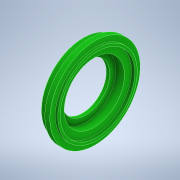
# Autodesk Inventor part: Крышка_Левая
Saved by Autodesk Inventor 2021 (Build 250183000, 183)
## iProperties
Created: 2023-04-24
Part Number: Крышка_Левая
Material: Сталь, углеродистая
Document SubType Name: Modeling
Designer: gdevc
Density: 7.85 g/cm^3
Appearance: Темно-зеленый
Author: gdevc
Autodesk Inventor part; units mm, degrees
ref_plane "YZ Plane" through (0, 0, 0) normal (1, 0, 0) x (0, 1, 0)
ref_plane "XZ Plane" through (0, 0, 0) normal (0, 1, 0) x (-1, 0, 0)
ref_plane "XY Plane" through (0, 0, 0) normal (0, 0, 1) x (1, 0, 0)
sketch "Эскиз1" plane through (0, 0, 0) normal (0, 0, 1) x (1, 0, 0)
  line L0 (0, 0) -> (118.4333, 0)
  line L1 (0, 28.5) -> (4, 28.5)
  line L2 (4, 28.5) -> (4, 36)
  line L3 (0, 28.5) -> (0, 50)
  line L4 (0, 50) -> (9, 50)
  line L5 (9, 50) -> (9, 54)
  line L6 (9, 54) -> (15, 54)
  line L7 (15, 54) -> (15, 47.5)
  line L8 (4, 36) -> (12, 36)
  line L9 (15, 47.5) -> (18, 47.5)
  line L10 (18, 47.5) -> (18, 44.5)
  line L11 (18, 44.5) -> (14.1429, 44.5)
  line L12 (14.1429, 44.5) -> (14.1429, 36)
  line L13 (14.1429, 36) -> (12, 36)
  dimension "d0" = 57
  dimension "d1" = 100
  dimension "d3" = 6
  dimension "d4" = 4
  dimension "d6" = 72
  dimension "d7" = 8
  dimension "d8" = 4
  dimension "d10" = 3
  dimension "d11" = 95
  dimension "d13" = 9
  dimension "d17" = 3
  constraints: 28 end point, 6 perpendicular, 4 horizontal, 2 vertical, 1 collinear, 1 point on line
  measures "d0" diameter of L1 L0
  measures "d1" diameter of L4 L0
  measures "d3" distance of L5.end L6.end
  measures "d4" distance between parallel lines of L4 L6
  measures "d6" diameter of L8 L0
  measures "d7" distance of L2.end L8.end
  measures "d8" distance between parallel lines of L3 L2
  measures "d10" distance of L7.end L9.end
  measures "d11" diameter of L9 L0
  measures "d13" distance of L3.end L4.end
  measures "d17" distance of L9.end L10.end
revolve "Вращение1" add sketch "Эскиз1" angle 360 about axis through (0, 0, 0) along (1, 0, 0)
chamfer "Фаска1" distance 1 angle 45 1 edges at (0, -50, 0)
